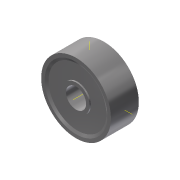
# Autodesk Inventor part: empty
Saved by Autodesk Inventor 2014 (Build 180170000, 170)
## iProperties
Created: 2015-04-13
Part Number: empty
Material: Generic
Document SubType Name: Modeling
Designer: Martin
Density: 1 g/cm^3
Appearance: Default
Author: Martin
Autodesk Inventor part; units mm, degrees
ref_plane "YZ Plane" through (0, 0, 0) normal (1, 0, 0) x (0, 1, 0)
ref_plane "XZ Plane" through (0, 0, 0) normal (0, 1, 0) x (-1, 0, 0)
ref_plane "XY Plane" through (0, 0, 0) normal (0, 0, 1) x (1, 0, 0)
sketch "Sketch1" plane through (0, 0, 0) normal (1, 0, 0) x (0, 1, 0)
  line L0 (0, -1) -> (0, 6) projected
  line L1 (-2.8, 0) -> (2.8, 0) projected
  line L2 (-2, 1.44) -> (2, 1.44)
  line L3 (2, 1.44) -> (2, 1.94)
  line L4 (2, 1.94) -> (1.8, 1.94)
  line L5 (1.8, 1.94) -> (1.8, 4.14)
  line L6 (1.8, 4.14) -> (2, 4.5)
  line L7 (2, 4.5) -> (2, 5)
  line L8 (2, 5) -> (-2, 5)
  line L9 (-2, 5) -> (-2, 4.5)
  line L10 (-2, 4.5) -> (-1.8, 4.14)
  line L11 (-1.8, 4.14) -> (-1.8, 1.94)
  line L12 (-1.8, 1.94) -> (-2, 1.94)
  line L13 (-2, 1.94) -> (-2, 1.44)
  point P0 (0, 0)
  dimension "d0" = 2.88
  dimension "d1" = 10
  dimension "d2" = 4
  dimension "d3" = 0.5
  dimension "d4" = 0.5
  dimension "d5" = 2.2
  dimension "d6" = 0.2
  constraints: 24 end point, 8 parallel, 2 collinear, 1 perpendicular, 5 other
  measures "d0" diameter of L2 L1
  measures "d1" diameter of L8 L1
  measures "d2" distance of L7.end L8.end
  measures "d3" distance of L12.end L2.start
  measures "d4" distance of L8.end L9.end
  measures "d5" distance of L10.end L11.end
  measures "d6" distance of L11.end L12.end
revolve "Revolution1" add sketch "Sketch1" angle 360 about axis through (0, -10, 0) along (0, 1, 0)
body "Solid1"
